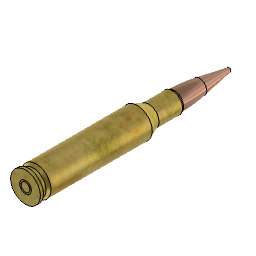
12-7x99mm_FMJ_mk1_v4 (Autodesk Fusion 360 design; units mm, degrees)
Autodesk Fusion 360 part; units mm, degrees
note: some values were not read from the file. Set by a fixed rule: which sketch regions a step uses.
sketch "スケッチ1" plane through (0, 0, 0) normal (0, 0, 1) x (1, 0, 0)
  line L0 (-10.2105, 0) -> (10.2105, 0)
  line L1 (0, 0) -> (0, 2.108) construction
  line L2 (-8.636, 2.108) -> (8.636, 2.108) construction
  line L3 (-10.2105, 0) -> (-10.2105, 2.108)
  line L4 (-10.2105, 2.108) -> (-8.636, 2.108)
  line L5 (-8.636, 2.108) -> (-8.636, 5.384)
  line L6 (-8.636, 5.384) -> (-10.2105, 7.2604)
  line L7 (-10.2105, 2.108) -> (-10.2105, 7.2604) construction
  line L8 (-10.2105, 7.2604) -> (-10.2105, 76.352)
  line L9 (-7.112, 100.2) -> (7.112, 100.2)
  line L10 (0, 0) -> (0, 100.2)
  line L11 (-7.112, 100.2) -> (-7.112, 84.097)
  line L12 (-7.112, 84.097) -> (-10.2105, 76.352)
  line L13 (-4.0005, 0) -> (-4.0005, 5.384)
  line L14 (4.0005, 0) -> (4.0005, 5.384)
  line L15 (-4.0005, 5.384) -> (4.0005, 5.384)
  line L16 (7.112, 100.2) -> (7.112, 84.097)
  line L17 (7.112, 84.097) -> (10.2105, 76.352)
  line L18 (10.2105, 7.2604) -> (10.2105, 76.352)
  line L19 (8.636, 5.384) -> (10.2105, 7.2604)
  line L20 (8.636, 2.108) -> (8.636, 5.384)
  line L21 (10.2105, 2.108) -> (8.636, 2.108)
  line L22 (10.2105, 0) -> (10.2105, 2.108)
  line L23 (-8.2105, 9.2604) -> (-8.2105, 75.9668)
  line L24 (-5.612, 82.462) -> (-8.2105, 75.9668)
  line L25 (-5.612, 100.2) -> (-5.612, 82.462)
  line L26 (5.612, 100.2) -> (5.612, 82.462)
  line L27 (5.612, 82.462) -> (8.2105, 75.9668)
  line L28 (8.2105, 9.2604) -> (8.2105, 75.9668)
  line L29 (-6.2105, 7.2604) -> (6.2105, 7.2604)
  arc A0 (-8.2105, 9.2604) -> (-6.2105, 7.2604) centre (-6.2105, 9.2604) ccw
  arc A1 (6.2105, 7.2604) -> (8.2105, 9.2604) centre (6.2105, 9.2604) ccw
  line L30 (0, 100.2) -> (0, 140)
  line L31 (-6.4895, 100.2) -> (-6.4895, 110.2)
  line L32 (6.4895, 100.2) -> (6.4895, 110.2)
  line L33 (-6.4895, 110.2) -> (6.4895, 110.2) construction
  circle A2 centre (0, 138.5) radius 1.5
  line L34 (-6.4895, 110.2) -> (-1.4774, 138.7593)
  line L35 (6.4895, 110.2) -> (1.4774, 138.7593)
  line L36 (-5.612, 82.462) -> (5.612, 82.462)
  dimension "d1" = 20.421
  dimension "d2" = 2.108
  dimension "d3" = 17.272
  dimension "d5" = 5.384
  dimension "d6" = 40
  dimension "d7" = 76.352
  dimension "d8" = 14.224
  dimension "d9" = 100.2
  dimension "d10" = 16.103
  dimension "d11" = 8.001
  dimension "d12" = 5.384
  dimension "d15" = 2
  dimension "d20" = 140
  dimension "d22" = 12.979
  dimension "d23" = 10
  dimension "d25" = 3
  constraint horizontal L0
  constraint midpoint L1.start L0
  constraint coincident L1.start L10.start
  constraint perpendicular L0 L1
  constraint horizontal L2
  constraint midpoint L1.end L2
  constraint perpendicular L0 L3
  constraint perpendicular L3 L4
  constraint perpendicular L2 L5
  constraint parallel L3 L7
  constraint parallel L7 L8
  constraint horizontal L9
  constraint midpoint L9 L10.end
  constraint perpendicular L0 L10
  constraint perpendicular L9 L11
  constraint coincident L0 L13.start
  constraint perpendicular L2 L13
  constraint coincident L0 L14.start
  constraint perpendicular L2 L14
  constraint perpendicular L14 L15
  constraint symmetric L0.start L10 L0.end
  constraint symmetric L2.start L10 L2.end
  constraint symmetric L3.end L10 L21.start
  constraint symmetric L5.end L10 L19.start
  constraint symmetric L6.end L10 L18.start
  constraint symmetric L8.end L10 L17.end
  constraint symmetric L9.start L10 L9.end
  constraint symmetric L10 L11.end L16.end
  constraint perpendicular L28 L29
  constraint tangent L23 A0
  constraint tangent L29 A0
  constraint tangent L28 A1
  constraint tangent L29 A1
  constraint equal A0 A1
  constraint perpendicular L9 L30
  constraint coincident L9 L31.start
  constraint perpendicular L9 L31
  constraint coincident L9 L32.start
  constraint perpendicular L9 L32
  constraint perpendicular L31 L33
  constraint symmetric L30 L31 L32
  constraint coincident L30.end A2
  constraint coincident A2 L34.end
  constraint tangent A2 L34
  constraint coincident A2 L35.end
  constraint tangent A2 L35
  measures "d1" distance of L0.start L0.end
  measures "d2" distance of L1.start L1.end
  measures "d3" distance of L2.start L2.end
  measures "d5" distance of L0 L5.end
  measures "d6" angle of L6 L7
  measures "d7" distance of L0.start L8.end
  measures "d8" distance of L9.start L9.end
  measures "d9" distance of L0 L9
  measures "d10" distance of L9.start L11.end
  measures "d11" distance of L13.end L14.end
  measures "d12" distance of L13.start L13.end
  measures "d15" radius of A0
  measures "d20" distance of L1.start L30.end
  measures "d22" distance of L31.end L32.end
  measures "d23" distance of L31.start L31.end
  measures "d25" diameter of A2
revolve "回転1" add sketch "スケッチ1" angle 360 about axis through (0, 0, 0) along (0, 1, 0) contours L0 L3 L4 L5 L6 L8 L9 L10 L11 L12 L13 L15 L23 L24 L25 L29 A0 makes body 1
revolve "回転2" add sketch "スケッチ1" angle 360 about axis through (0, 0, 0) along (0, 1, 0) separate body contours L0 L10 L13 L15 makes body 2
fillet "フィレット1" radius 1 1 edges at (-3.7298, 0, 1.4466) on bodies 2
combine "結合1" operation add target body 2 tool bodies 1
revolve "回転3" add sketch "スケッチ1" angle 360 about axis through (0, 100.2, 0) along (0, 1, 0) separate body contours L9 L10 L25 L36 | L9 L30 L31 A2 L34 | L30 A2 picked at (0.5207, 138.724) makes body 3
fillet "フィレット2" radius 100 1 edges at (-6.0503, 110.2, 2.3467) on bodies 3
move_face "面をオフセット1" offset -0.2 1 faces at (-5.5841, 88.3747, -0.5588) on bodies 3
equation "d12 = d5"
